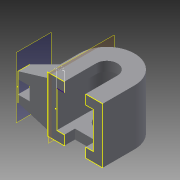
# Autodesk Inventor part: 零件6-22
Saved by Autodesk Inventor 2014 (Build 180170000, 170)
## iProperties
Created: 2018-11-23
Part Number: 零件6-22
Material: 常规
Document SubType Name: 钣金
Designer: Administrator
Density: 1 g/cm^3
Sheet Metal Rule: 默认
Appearance: 默认
Author: Administrator
Autodesk Inventor part; units mm, degrees
ref_plane "XZ Plane" through (0, 0, 0) normal (0, 1, 0) x (-1, 0, 0)
ref_plane "XY Plane" through (0, 0, 0) normal (0, 0, 1) x (1, 0, 0)
sketch "草图1" plane through (0, 0, 0) normal (0, 1, 0) x (-1, 0, 0)
  line L0 (234.2186, 0) -> (-293.6058, 0)
  line L1 (7.25, 23.5) -> (-7.25, 23.5)
  line L2 (-7.25, -23.5) -> (7.25, -23.5)
  line L3 (7.25, -23.5) -> (7.25, 23.5)
  line L4 (7.25, 23.5) -> (-7.25, -23.5) construction
  line L5 (-7.25, 23.5) -> (7.25, -23.5) construction
  line L6 (-7.25, 15.5) -> (-0.75, 15.5)
  line L7 (-0.75, 15.5) -> (-0.75, -15.5)
  line L8 (-0.75, -15.5) -> (-7.25, -15.5)
  line L9 (-13.75, 15.5) -> (-0.75, -15.5) construction
  line L10 (-0.75, 15.5) -> (-13.75, -15.5) construction
  line L11 (-7.25, 23.5) -> (-7.25, 15.5)
  line L12 (-7.25, -15.5) -> (-7.25, -23.5)
  point P0 (0, 0)
  point P1 (-7.25, 0)
  dimension "d0" = 14.5
  dimension "d1" = 47
  dimension "d2" = 13
  constraints: 26 end point, 4 midpoint, 4 parallel, 3 horizontal, 3 perpendicular
  measures "d0" distance of L2.end L2.start
  measures "d1" distance of L1.end L2.start
  measures "d2" distance of L7.end L10.end
sketch "草图2" plane through (0, 0, 0) normal (0, 1, 0) x (-1, 0, 0)
  point P0 (0, 0)
sketch "草图3" plane through (0, 0, 0) normal (0, 0, 1) x (1, 0, 0)
  line L0 (0, 0) -> (0, 27)
  arc A0 (32.5, 27) -> (0, 27) centre (16.25, 27) ccw
  line L1 (32.5, 27) -> (32.5, 0)
  dimension "d4" = 27
  dimension "d5" = 32.5
  constraints: 4 end point, 2 point on circle, 1 centre point, 1 parallel, 1 tangent, 1 vertical
  measures "d4" distance of L0.start L0.end
  measures "d5" diameter of A0
sweep "扫掠1" add profiles "草图1" path "草图3"
sketch "草图4" plane through (7.25, 0, -23.5) normal (0, 0, -1) x (-1, 0, 0)
  line L0 (-18, 27) -> (-18, 0) projected
  arc A0 (0, 27) -> (-18, 27) centre (-9, 27) ccw projected
  line L1 (0, 0) -> (0, 27) projected
  arc A1 (-18, 27) -> (0, 27) centre (-9, 27) ccw
  line L2 (-18, 9) -> (0, 9)
  line L3 (-18, 9) -> (-18, 27)
  line L4 (0, 9) -> (0, 27)
  point P0 (7.25, 0)
  dimension "d7" = 18
  constraints: 6 end point, 4 tangent, 2 collinear, 2 point on circle, 2 point on line, 1 centre point, 1 coincident, 1 concentric, 1 perpendicular
  measures "d7" distance from line of L2 A1.centre
extrude "拉伸1" add sketch "草图4" against normal blind 8 contours A1 L1 L2 L0
sketch "草图5" plane through (-7.25, 0, 23.5) normal (0, -1, 0) x (1, 0, 0)
  line L0 (0, 0) -> (14.5, 0) projected
  line L1 (0, -47) -> (0, 0) projected
  line L2 (14.5, -47) -> (0, -47) projected
  line L3 (14.5, -39) -> (14.5, -47) projected
  line L4 (8, -39) -> (14.5, -39) projected
  line L5 (8, -8) -> (8, -39) projected
  line L6 (14.5, -8) -> (8, -8) projected
  line L7 (14.5, 0) -> (14.5, -8) projected
  point P0 (7.25, -23.5)
sketch "草图6" plane through (25.25, 0, 23.5) normal (0, -1, 0) x (1, 0, 0)
  line L0 (14.5, 0) -> (0, 0) projected
  line L1 (0, 0) -> (0, -8) projected
  line L2 (0, -8) -> (6.5, -8) projected
  line L3 (6.5, -8) -> (6.5, -39) projected
  line L4 (6.5, -39) -> (0, -39) projected
  line L5 (0, -39) -> (0, -47) projected
  line L6 (0, -47) -> (14.5, -47) projected
  line L7 (14.5, -47) -> (14.5, 0) projected
  point P0 (-25.25, -23.5)
sketch "草图7" plane through (-7.25, 0, 23.5) normal (0, -1, 0) x (1, 0, 0)
  line L0 (0, 0) -> (14.5, 0) projected
  line L1 (0, -47) -> (0, 0) projected
  line L2 (14.5, -47) -> (0, -47) projected
  line L3 (14.5, -39) -> (14.5, -47) projected
  line L4 (8, -39) -> (14.5, -39) projected
  line L5 (8, -8) -> (8, -39) projected
  line L6 (14.5, -8) -> (8, -8)
  line L7 (14.5, 0) -> (14.5, -8) projected
  point P0 (7.25, -23.5)
  dimension "d10" = 6.5
  constraints: 2 end point
  measures "d10" distance of L6.start L5.start
sketch "草图8" plane through (-7.25, 0, 23.5) normal (0, -1, 0) x (1, 0, 0)
  line L0 (8, -8) -> (8, -39) projected
  circle A0 centre (23.5, -23.5) radius 9
  point P0 (7.25, -23.5)
  dimension "d11" = 18
  dimension "d12" = 15.5
  constraints: 1 centre point
  measures "d11" diameter of A0
  measures "d12" distance from line of A0.centre L0
extrude "拉伸2" cut sketch "草图8" against normal blind 232
sketch "草图9" plane through (-7.25, 0, -23.5) normal (-1, 0, 0) x (0, 0, 1)
  line L0 (42.5, 0) -> (4.5, 0)
  line L1 (4.5, 0) -> (4.5, 20)
  line L2 (4.5, 20) -> (42.5, 20)
  line L3 (42.5, 20) -> (42.5, 0)
  line L4 (42.5, 0) -> (4.5, 20) construction
  line L5 (4.5, 0) -> (42.5, 20) construction
  line L6 (47, 0) -> (39, 0) projected
  point P0 (23.5, 0)
  point P1 (23.5, 10)
  point P2 (43, 0)
  dimension "d15" = 38
  dimension "d16" = 20
  constraints: 12 end point, 3 midpoint, 2 parallel, 1 horizontal, 1 perpendicular, 1 point on line
  measures "d15" distance of L1.end L2.end
  measures "d16" distance of L0.end L1.end
ref_plane "工作平面1" through (-3.625, 0, 0) normal (1, 0, 0) x (0, 1, 0)
ref_plane "工作平面2" through (-32.25, 0, -23.5) normal (-1, 0, 0) x (0, 0, 1)
sketch "草图10" plane through (-32.25, 0, -23.5) normal (-1, 0, 0) x (0, 0, 1)
  line L0 (12, 0) -> (35, 0)
  line L1 (35, 0) -> (35, 10)
  line L2 (35, 10) -> (12, 10)
  line L3 (12, 10) -> (12, 0)
  line L4 (12, 0) -> (35, 10) construction
  line L5 (35, 0) -> (12, 10) construction
  point P0 (23.5, 0)
  point P1 (23.5, 5)
  point P2 (39, 0)
  dimension "d18" = 23
  dimension "d19" = 10
  constraints: 12 end point, 2 midpoint, 2 parallel, 1 horizontal, 1 perpendicular, 1 point on line
  measures "d18" distance of L2.end L1.end
  measures "d19" distance of L0.end L1.end
loft "放样1" add profiles "草图10", "草图9"
sketch "草图11" plane through (-32.25, 0, 11.5) normal (-1, 0, 0) x (0, 0, 1)
  line L0 (-23, 0) -> (0, 0) projected
  line L1 (0, 0) -> (0, 10) projected
  line L2 (0, 10) -> (-23, 10) projected
  line L3 (-23, 10) -> (-23, 0) projected
  point P0 (-11.5, 0)
sketch "草图12" plane through (-7.25, 0, 23.5) normal (0, -1, 0) x (1, 0, 0)
  line L0 (-25, -35) -> (-25, -12) projected
  line L1 (-15, -29.113) -> (-25, -29.113)
  line L2 (-25, -29.113) -> (-25, -17.887)
  line L3 (-25, -17.887) -> (-15, -17.887)
  line L4 (-15, -17.887) -> (-15, -29.113)
  line L5 (-15, -29.113) -> (-25, -17.887) construction
  line L6 (-25, -29.113) -> (-15, -17.887) construction
  point P0 (7.25, -23.5)
  point P1 (-20, -23.5)
  point P2 (-25, -23.5)
  dimension "d24" = 10
  constraints: 12 end point, 4 midpoint, 2 parallel, 1 horizontal, 1 perpendicular
  measures "d24" distance of L2.end L3.end
extrude "拉伸3" cut sketch "草图12" against normal blind 232
equation "\"折弯半径\" = 厚度"
equation "\"折弯释压宽度\" = 厚度"
equation "\"折弯释压深度\" = 0.5 * 厚度"
equation "\"拐角释压尺寸\" = 4 * 厚度"
equation "\"最小余量\" = 2 * 厚度"
equation "\"过渡半径\" = 折弯半径"
equation "\"Jacobi半径尺寸\" = 厚度"
equation "\"间隙大小\" = 厚度"
equation "\"厚度\" = 0.5"
